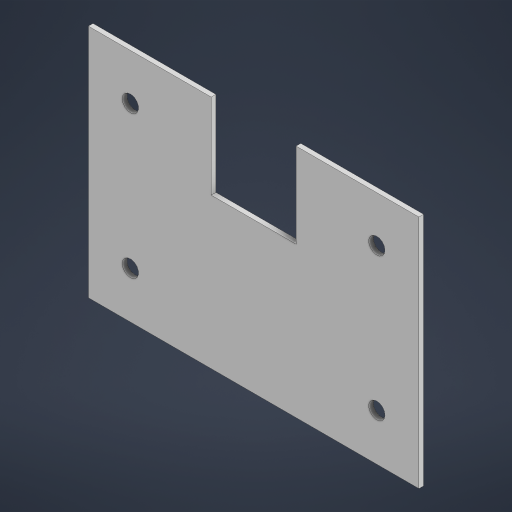
# Autodesk Inventor part: DIFF_HOUSING_NO
Saved by Autodesk Inventor 2024 (Build 280153000, 153)
## iProperties
Created: 2024-01-10
Part Number: DIFF_HOUSING_NO
Material: Generic
Document SubType Name: Modeling
Designer: bugme
Density: 1 g/cm^3
Appearance: Default
Author: bugme
Autodesk Inventor part; units mm, degrees
ref_plane "YZ Plane" through (0, 0, 0) normal (1, 0, 0) x (0, 1, 0)
ref_plane "XZ Plane" through (0, 0, 0) normal (0, 1, 0) x (-1, 0, 0)
ref_plane "XY Plane" through (0, 0, 0) normal (0, 0, 1) x (1, 0, 0)
sketch "Sketch1" plane through (0, 0, 0) normal (0, 0, 1) x (1, 0, 0)
  line L0 (-55.88, 39.751) -> (-55.88, -39.751)
  line L1 (-55.88, 39.751) -> (23.622, 39.751) construction
  line L2 (-55.88, -39.751) -> (55.88, -39.751)
  line L3 (55.88, -39.751) -> (55.88, 39.751)
  line L4 (55.88, 39.751) -> (-55.88, 39.751)
  line L5 (0, -55.6514) -> (0, 55.6514) projected
  line L6 (-78.232, 0) -> (78.232, 0) projected
  line L7 (-14.351, 39.751) -> (-14.351, 11.049)
  line L8 (-14.351, 11.049) -> (14.351, 11.049)
  line L9 (14.351, 11.049) -> (14.351, 39.751)
  point P0 (0, 0)
  dimension "d0" = 79.502
  dimension "d1" = 90
  dimension "d2" = 111.76
  dimension "d3" = 28.702
  dimension "d4" = 28.702
  constraints: 16 end point, 7 perpendicular, 2 point on line, 1 horizontal, 1 vertical, 3 other
  measures "d0" distance of L0.start L0.end
  measures "d1" angle of L0 L1
  measures "d2" distance of L0.end L2.end
  measures "d3" distance of L7.start L7.end
  measures "d4" distance of L7.end L8.end
extrude "Extrusion1" add sketch "Sketch1" along normal blind 1.5875 contours L4 L7 L8 L5 L6 L0 | L6 L5 L2 L0 | L6 L3 L2 L5 | L5 L8 L9 L4 L3 L6
sketch "Sketch2" plane through (-41.656, -2.7227, 1.5875) normal (0, 0, 1) x (1, 0, 0)
  line L0 (97.536, -37.0283) -> (97.536, 37.0283)
  line L1 (-14.224, -37.0283) -> (97.536, -37.0283)
  line L2 (97.536, -37.0283) -> (97.536, 42.4737) projected
  line L3 (-14.224, -37.0283) -> (97.536, -37.0283) projected
  point P0 (0, 0)
  point P1 (83.312, 26.9797)
  point P2 (83.312, -21.2803)
  point P3 (97.536, 0)
  point P4 (41.656, -37.0283)
  dimension "d10" = 48.26
  dimension "d11" = 14.224
  dimension "d9" = 14.224
  dimension "d8" = 15.748
  constraints: 4 end point, 3 midpoint, 1 point on line
  measures "d10" distance of point (83.312, -21.28) point (83.312, 26.98)
  measures "d11" distance from line of L0 point (83.312, 26.98)
  measures "d9" distance from line of L0 point (83.312, -21.28)
  measures "d8" distance from line of L1 point (83.312, -21.28)
hole "Hole1" at (41.656, 24.257, 1.5875) at (41.656, -24.003, 1.5875) direction (0, 0, -1) diameter 5.5118 end through all
mirror "Mirror1" about plane through (0, 0, 0) normal (1, 0, 0) of "Hole1"
body "Solid1"
